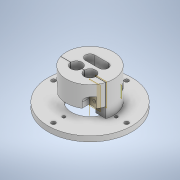
# Autodesk Inventor part: big_actuator_holder
Saved by Autodesk Inventor 2021 (Build 250183000, 183)
## iProperties
Created: 2020-10-24
Part Number: big_actuator_holder
Material: Generic
Document SubType Name: Modeling
Designer: bober
Density: 1 g/cm^3
Appearance: Default
Author: bober
Autodesk Inventor part; units mm, degrees
ref_plane "YZ Plane" through (0, 0, 0) normal (1, 0, 0) x (0, 1, 0)
ref_plane "XZ Plane" through (0, 0, 0) normal (0, 1, 0) x (-1, 0, 0)
ref_plane "XY Plane" through (0, 0, 0) normal (0, 0, 1) x (1, 0, 0)
sketch "Sketch1" plane through (0, 0, 0) normal (0, 1, 0) x (-1, 0, 0)
  line L0 (-6.5, 6.5) -> (6.5, 6.5)
  line L1 (6.5, 6.5) -> (6.5, -6.5)
  line L2 (6.5, -6.5) -> (-6.5, -6.5)
  line L3 (-6.5, -6.5) -> (-6.5, 6.5)
  line L4 (-6.5, 6.5) -> (6.5, -6.5) construction
  line L5 (6.5, 6.5) -> (-6.5, -6.5) construction
  circle A0 centre (6.5, 6.5) radius 5.45
  circle A1 centre (-6.5, 6.5) radius 5.45
  line L6 (6.5, -6.5) -> (-6.5, -6.5) construction
  line L7 (6.5, -2) -> (-6.5, -2)
  line L8 (-6.5, -11) -> (6.5, -11)
  arc A2 (6.5, -11) -> (6.5, -2) centre (6.5, -6.5) ccw
  arc A3 (-6.5, -2) -> (-6.5, -11) centre (-6.5, -6.5) ccw
  circle A4 centre (0, 0) radius 22.5
  line L9 (-23.5, 6.6) -> (36.5, 6.6)
  line L10 (36.5, 6.6) -> (36.5, 6.4)
  line L11 (36.5, 6.4) -> (-23.5, 6.4)
  line L12 (-23.5, 6.4) -> (-23.5, 6.6)
  line L13 (-23.5, 6.6) -> (36.5, 6.4) construction
  line L14 (36.5, 6.6) -> (-23.5, 6.4) construction
  point P0 (0, -6.5)
  point P1 (11.9491, 6.6)
  point P2 (21.5102, 6.6)
  point P3 (-21.5102, 6.6)
  point P4 (-11.9491, 6.6)
  point P5 (-1.0509, 6.6)
  point P6 (1.0509, 6.6)
  point P7 (1.0509, 6.4)
  point P8 (-1.0509, 6.4)
  point P9 (-11.9491, 6.4)
  point P10 (-21.5706, 6.4)
  point P11 (21.5706, 6.4)
  point P12 (11.9491, 6.4)
  dimension "d0" = 13
  dimension "d1" = 13
  dimension "d2" = 10.9
  dimension "d3" = 10.9
  dimension "d4" = 9
  dimension "d5" = 45
  dimension "d6" = 60
  dimension "d7" = 0.2
  constraints: 32 end point, 5 centre point, 5 midpoint, 5 parallel, 4 coincident, 4 point on circle, 4 tangent, 3 horizontal, 2 perpendicular
  measures "d0" distance of L1.end L2.end
  measures "d1" distance of L0.end L1.end
  measures "d2" diameter of A0
  measures "d3" diameter of A1
  measures "d4" diameter of A3
  measures "d5" diameter of A4
  measures "d6" distance of L10.end L11.end
  measures "d7" distance of L9.end L10.end
extrude "Extrusion1" add sketch "Sketch1" along normal blind 20 contours A1 L9 A4 A0 | L11 A0 L1 L7 L3 A1 | L3 A3 L8 A2 L1 A0 L11 A4 A1
extrude "Extrusion2" add sketch "Sketch1" against normal blind 10 contours L11 A0 L1 L7 L3 A1 | L3 A3 L8 A2 L1 A0 L11 A4 A1
sketch "Sketch2" plane through (0, -10, 0) normal (0, -1, 0) x (1, 0, 0)
  circle A0 centre (0, 0) radius 17.5
  circle A1 centre (0, 0) radius 40
  dimension "d12" = 35
  dimension "d13" = 80
  constraints: 2 centre point, 2 coincident
  measures "d12" diameter of A0
  measures "d13" diameter of A1
extrude "Extrusion3" add sketch "Sketch2" along normal blind 5
sketch "Sketch3" plane through (0, -10, 0) normal (0, 1, 0) x (1, 0, 0)
  circle A0 centre (0, 25) radius 1.5
  circle A1 centre (0, 35) radius 2
  point P0 (0, 0)
  dimension "d16" = 3
  dimension "d44" = 4
  constraints: 2 centre point
  measures "d16" diameter of A0
  measures "d44" diameter of A1
extrude "Extrusion4" cut sketch "Sketch3" against normal blind 5
pattern_circular "Circular Pattern1" count 4 over 360 about axis through (0, -10, 0) along (0, -1, 0) of "Extrusion4"
sketch "Sketch4" plane through (21.5102, 0, 6.6) normal (0, 0, -1) x (-1, 0, 0)
  circle A0 centre (4.8812, 5) radius 1.5
  point P0 (21.5102, 0)
  dimension "d22" = 3
  constraints: 1 centre point
  measures "d22" diameter of A0
extrude "Extrusion5" cut sketch "Sketch4" along normal blind 30 and the other way blind 15
ref_plane "Work Plane1" through (21.5102, 0, -8.4) normal (0, 0, -1) x (-1, 0, 0)
sketch "Sketch5" plane through (21.5102, 0, -8.4) normal (0, 0, -1) x (-1, 0, 0)
  circle A0 centre (4.8812, 5) radius 1.5 projected
  circle A1 centre (4.8812, 5) radius 2.75
  line L0 (2.1312, 6.5877) -> (4.8812, 8.1754)
  line L1 (4.8812, 8.1754) -> (7.6312, 6.5877)
  line L2 (7.6312, 6.5877) -> (7.6312, 3.4123)
  line L3 (7.6312, 3.4123) -> (4.8812, 1.8246)
  line L4 (4.8812, 1.8246) -> (2.1312, 3.4123)
  line L5 (2.1312, 3.4123) -> (2.1312, 6.5877)
  point P0 (21.5102, 0)
  point P1 (2.1312, 5)
  dimension "d28" = 5.5
  constraints: 12 end point, 2 coincident, 1 horizontal alignment, 1 midpoint, 15 other
extrude "Extrusion6" cut sketch "Sketch5" along normal blind 30 contours A0 | A1 | L2 L3 A1 | A1 L1 L2 | A1 L0 L1 | L3 L4 A1 | A1 L5 L0 | L4 L5 A1
mirror "Mirror1" about plane through (0, 0, 0) normal (1, 0, 0) of "Extrusion6", "Extrusion5"
ref_plane "Work Plane2" through (11.9491, 20, 6.4) normal (0, 0, 1) x (1, 0, 0)
ref_plane "Work Plane3" through (11.9491, 20, 12.4) normal (0, 0, 1) x (1, 0, 0)
sketch "Sketch11" plane through (11.9491, 20, 12.4) normal (0, 0, 1) x (1, 0, 0)
  circle A0 centre (4.6799, -15) radius 1.5 projected
  circle A1 centre (4.6799, -15) radius 5
  line L0 (9.5611, -20) -> (-33.4593, -20) projected
  circle A2 centre (-28.5781, -15) radius 1.5 projected
  circle A3 centre (-28.5781, -15) radius 5
  line L1 (9.5611, -20) -> (-0.3201, -20)
  line L2 (-0.3201, -20) -> (-0.3201, -15)
  line L3 (-0.3201, -15) -> (9.5611, -15)
  line L4 (9.5611, -15) -> (9.5611, -20)
  line L5 (-33.4593, -20) -> (-33.4593, 0) projected
  line L6 (-33.4593, -20) -> (-23.5781, -20)
  line L7 (-23.5781, -20) -> (-23.5781, -15)
  line L8 (-23.5781, -15) -> (-33.4593, -15)
  line L9 (-33.4593, -15) -> (-33.4593, -20)
  point P0 (-11.9491, -20)
  point P1 (-30.0781, -15)
  point P2 (-27.0781, -15)
  point P3 (-33.4593, -16.0833)
  point P4 (-23.5781, -20)
  point P5 (9.5611, -16.0833)
  point P6 (-0.3201, -20)
  constraints: 16 end point, 4 horizontal, 4 parallel, 2 coincident, 2 perpendicular, 1 point on line, 6 other
extrude "Extrusion9" cut sketch "Sketch11" along normal blind 10 contours L3 L4 A1 A0 | A0 L3 A1 L4 | A1 L0 L2 | L4 L0 A1 | L0 A3 L7 | L0 L5 A3 | A3 L5 L8 A2 | L8 A2 L5 A3 | A3 L5 | A2 L8 picked at (-28.1208, -15.352)
sketch "Sketch12" plane through (0, -10, 0) normal (0, -1, 0) x (1, 0, 0)
  arc A0 (-11.9491, 6.4) -> (-1.0509, 6.4) centre (-6.5, 6.5) ccw projected
  line L0 (-6.5, 1.05) -> (6.527, 1.05)
  line L1 (6.527, 1.05) -> (6.527, 6.4)
  line L2 (6.527, 6.4) -> (-6.5, 6.4)
  line L3 (-6.5, 6.4) -> (-6.5, 1.05)
  point P0 (0, 0)
  point P1 (-1.0509, 6.4)
  constraints: 8 end point, 2 parallel, 1 horizontal, 1 perpendicular, 1 point on circle
extrude "Extrusion10" cut sketch "Sketch12" against normal blind 10 contours A0 L2 L1 L0
sketch "Sketch13" plane through (0, 0, 0) normal (1, 0, 0) x (0, 1, 0)
  line L0 (-2.4298, 26.0667) -> (21.3859, 26.0667)
  line L1 (21.3859, 26.0667) -> (21.3859, 6.4953)
  line L2 (21.3859, 6.4953) -> (-2.4298, 6.4953)
  line L3 (-2.4298, 6.4953) -> (-2.4298, 26.0667)
  point P0 (0, 0)
  constraints: 8 end point, 2 parallel, 1 horizontal, 1 perpendicular
split body "Split3" sketch "Sketch13" result two bodies curves L3 L0 L1 L2 first body at (-24.9233, -14.5, 10.0849)
body "Solid6"
body "Solid7"
